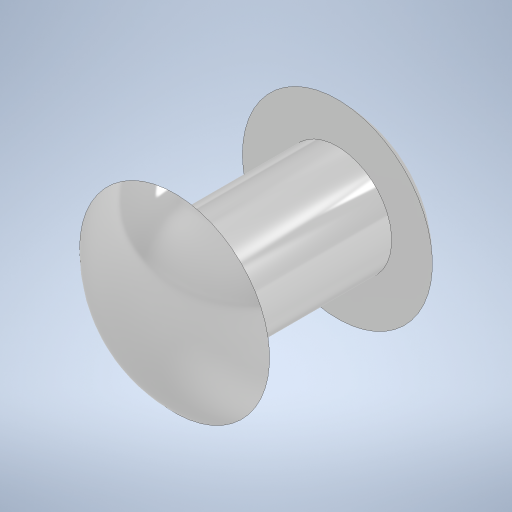
# Autodesk Inventor part: Rivet
Saved by Autodesk Inventor 2024 (Build 280153000, 153)
## iProperties
Created: 2021-04-22
Part Number: Rivet
Material: Aluminum 6061-AHC
Document SubType Name: Modeling
Designer: SauliusD
Density: 2.7 g/cm^3
Appearance: Aluminum - Dark
Author: SauliusD
Autodesk Inventor part; units mm, degrees
ref_plane "YZ Plane" through (0, 0, 0) normal (1, 0, 0) x (0, 1, 0)
ref_plane "XZ Plane" through (0, 0, 0) normal (0, 1, 0) x (-1, 0, 0)
ref_plane "XY Plane" through (0, 0, 0) normal (0, 0, 1) x (1, 0, 0)
sketch "Sketch1" plane through (0, 0, 0) normal (0, 0, 1) x (1, 0, 0)
  line L0 (0, 0) -> (-4, 0)
  line L1 (-4, 0) -> (-4, 12)
  line L2 (-4, 12) -> (0, 12)
  line L3 (0, 12) -> (0, 0)
  line L4 (-4, 12) -> (-7, 12)
  arc A0 (0, 15) -> (-7, 12) centre (0, 5.3333) ccw
  line L5 (0, 12) -> (0, 15)
  line L6 (-4, 6) -> (0, 6) construction
  line L7 (-4, 0) -> (0, 0)
  line L8 (-4, 0) -> (-7, 0)
  arc A1 (-7, 0) -> (0, -3) centre (0, 6.6667) ccw
  line L9 (0, 0) -> (0, -3)
  dimension "d1" = 12
  dimension "d2" = 3
  dimension "d3" = 8
  dimension "d4" = 14
  constraints: 20 end point, 4 point on circle, 3 symmetric about line, 2 centre point, 2 horizontal, 2 midpoint, 2 parallel, 1 perpendicular, 1 point on line, 1 vertical, 1 other
  measures "d1" distance of L0.end L1.end
  measures "d2" distance from line of L2 L5.end
  measures "d3" diameter of L1 L3
  measures "d4" diameter of L4.end L3
revolve "Revolution1" add sketch "Sketch1" angle 360 about axis through (0, 12, 0) along (0, -1, 0)
body "Solid1"
